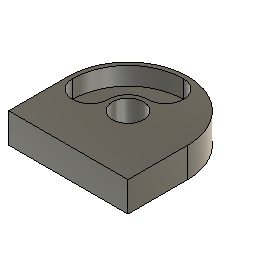
Support arm left printer attachment final v6 (Autodesk Fusion 360 archive; units mm, degrees)
design "Alternate hindge stop left"
Autodesk Fusion 360 part; units mm, degrees
sketch "Sketch1" plane through (0, 0, 0) normal (0, 0, 1) x (1, 0, 0)
  line L0 (0, 0) -> (20, 0)
  line L1 (0, 0) -> (0, 10)
  line L2 (20, 0) -> (20, 10)
  line L3 (0, 10) -> (20, 10) construction
  arc A0 (20, 10) -> (0, 10) centre (10, 10) ccw
  circle A1 centre (10, 10) radius 2.6
  dimension "d1" = 20
  dimension "d2" = 10
  dimension "d3" = 10
  dimension "d4" = 5.2
  constraint coincident L0.start L1.start
  constraint horizontal L0
  constraint perpendicular L0 L1
  constraint perpendicular L0 L2
  constraint midpoint L3 A0.centre
  constraint concentric A0 A1
  measures "d1" distance of L0.start L0.end
  measures "d2" distance of L0.start L1.end
  measures "d3" distance of L0.end L2.end
  measures "d4" diameter of A1
extrude "Extrude1" add sketch "Sketch1" along normal blind 5
sketch "Sketch2" plane through (0, 0, 5) normal (0, 0, 1) x (-1, 0, 0)
  circle A0 centre (-10, -10) radius 2.6
  line L0 (0, 0) -> (-20, 0)
  line L1 (-20, 0) -> (-20, -10)
  arc A1 (-20, -10) -> (0, -10) centre (-10, -10) ccw
  line L2 (0, -10) -> (0, 0)
  line L3 (-10, -10) -> (-10, -20) construction
  line L4 (-10, -10) -> (0, -10) construction
  arc A2 (-10, -13.3) -> (-6.7, -10) centre (-10, -10) ccw
  arc A3 (-10, -19.3) -> (-0.7, -10) centre (-10, -10) ccw
  line L5 (-0.7, -10) -> (-6.7, -10) construction
  line L6 (-10, -19.3) -> (-10, -13.3) construction
  arc A4 (-10, -13.3) -> (-10, -19.3) centre (-10, -16.3) ccw
  arc A5 (-0.7, -10) -> (-6.7, -10) centre (-3.7, -10) ccw
  dimension "d11" = 6.3
  dimension "d12" = 3
  constraint coincident A0.centre A1.centre
  constraint midpoint A1 L3.end
  constraint coincident A1.end L2.start
  constraint coincident L3 A2.start
  constraint coincident L4 A2.end
  constraint coincident L3 A3.start
  constraint coincident L4 A3.end
  constraint midpoint L6 A4.centre
  constraint midpoint L5 A5.centre
  measures "d11" distance of A0.centre A4.centre
  measures "d12" radius of A4
extrude "Extrude2" cut sketch "Sketch2" against normal blind 3 contours A2 A3 A4 A5
